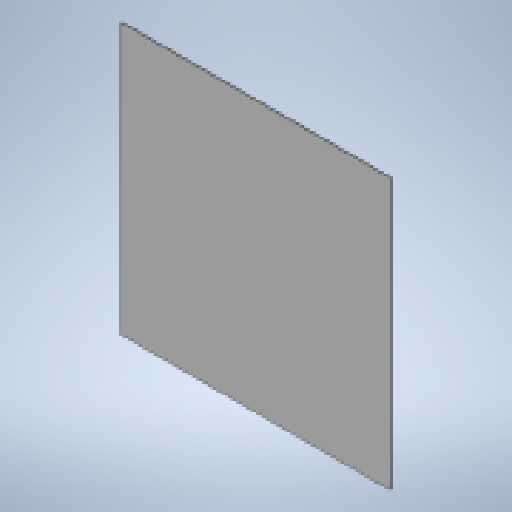
# Autodesk Inventor part: GBK 1111 shield 1
Saved by Autodesk Inventor 2026.2 (Build 302298000, 298)
## iProperties
Created: 2026-04-17
Part Number: GBK 1111 shield 1
Material: Steel
Document SubType Name: Sheet Metal
Designer: admin
Density: 7.85 g/cm^3
Sheet Metal Rule: Default_mm
Appearance: Default
Mass: 69243.3 g
Surface Area: 44341.6 cm^2
Volume: 8820.8 cm^3
Flat Pattern Width: 148 cm
Flat Pattern Length: 149 cm
Flat Pattern Area: 22052 cm^2
Sheet Metal Width: 1480,000 mm
Sheet Metal Length: 1490,000 mm
Sheet Metal Area: 2205200,000 mm^2
Stock Number: 1115
Author: admin
Autodesk Inventor part; units mm, degrees
ref_plane "YZ Plane" through (0, 0, 0) normal (1, 0, 0) x (0, 1, 0)
ref_plane "XZ Plane" through (0, 0, 0) normal (0, 1, 0) x (-1, 0, 0)
ref_plane "XY Plane" through (0, 0, 0) normal (0, 0, 1) x (1, 0, 0)
sketch "Sketch1" plane through (0, 0, 0) normal (0, 0, 1) x (1, 0, 0)
  line L0 (740, -745) -> (-740, -745)
  line L1 (-740, -745) -> (-740, 745)
  line L2 (-740, 745) -> (740, 745)
  line L3 (740, 745) -> (740, -745)
  line L4 (740, -745) -> (-740, 745) construction
  line L5 (-740, -745) -> (740, 745) construction
  point P0 (0, 0)
  dimension "d0" = 1480
  dimension "d1" = 1490
  measures "d0" distance of L1.end L2.end
  measures "d1" distance of L0.end L1.end
extrude "Plate1" add sketch "Sketch1" along normal blind 4
sketch "Sketch3" plane through (0, 0, 0) normal (0, 0, -1) x (-1, 0, 0)
  line L0 (-363.6739, -491) -> (-320.6849, -491) projected
  line L1 (-363.6739, 5.6667) -> (-320.6849, 5.6667) projected
  line L2 (-363.6739, 502.3333) -> (-320.6849, 502.3333) projected
  line L3 (-738.6395, 502.3333) -> (-680, 502.3333) projected
  line L4 (-738.6395, 5.6667) -> (-680, 5.6667) projected
  line L5 (-738.6395, -491) -> (-680, -491) projected
  line L6 (710, -491) -> (770, -491) projected
  line L7 (710, 5.6667) -> (770, 5.6667) projected
  line L8 (710, 502.3333) -> (770, 502.3333) projected
  line L9 (518.4821, 445.8246) -> (518.4821, 83.8729) construction
  line L10 (518.4821, 83.8729) -> (433.3265, 83.8729) construction
  line L11 (433.3265, 83.8729) -> (433.3265, 445.8246) construction
  line L12 (433.3265, 445.8246) -> (518.4821, 445.8246) construction
  line L13 (689.8679, -494.5) -> (689.8679, -591.5) projected
  line L14 (189.7393, -494.5) -> (189.7393, -591.5) projected
  line L15 (-310.3893, -494.5) -> (-310.3893, -591.5) projected
  ellipse E0 centre (-310.3893, 743.5) end of major axis (-310.3893, 773.5) minor radius 0.6803 (-310.3893, 713.5) -> (-310.3893, 773.5) ccw projected
  ellipse E1 centre (189.7393, 743.5) end of major axis (189.7393, 773.5) minor radius 0.6803 (189.7393, 713.5) -> (189.7393, 773.5) ccw projected
  ellipse E2 centre (689.8679, 743.5) end of major axis (689.8679, 773.5) minor radius 0.6803 (689.8679, 713.5) -> (689.8679, 773.5) ccw projected
  point P0 (0, 0)
  constraints: 8 other
mark "Mark2"
equation "\"d0\" = Лист_ширина"
equation "\"d1\" = 0.5 * Лист_длина"
equation "\"d2\" = Thickness"
equation "\"BendRadius\" = Thickness"
equation "\"BendReliefWidth\" = Thickness"
equation "\"BendReliefDepth\" = 0.5 * Thickness"
equation "\"CornerReliefSize\" = 4 * Thickness"
equation "\"MinimumRemnant\" = 2 * Thickness"
equation "\"TransitionRadius\" = BendRadius"
equation "\"JacobiRadiusSize\" = BendRadius"
equation "\"GapSize\" = Thickness"
equation "\"Лист_ширина\" = 1480"
equation "\"Лист_длина\" = 2980"
equation "\"Thickness\" = 4"
body "Solid1"
